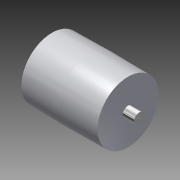
# Autodesk Inventor part: Flexiwheel Roller
Saved by Autodesk Inventor 2014 (Build 180170000, 170)
## iProperties
Created: 2014-02-03
Part Number: Flexiwheel Roller
Material: PPS Plastic
Document SubType Name: Modeling
Designer: Spooner
Density: 1.637 g/cm^3
Appearance: Snow
Author: Spooner
Autodesk Inventor part; units mm, degrees
ref_plane "YZ Plane" through (0, 0, 0) normal (1, 0, 0) x (0, 1, 0)
ref_plane "XZ Plane" through (0, 0, 0) normal (0, 1, 0) x (-1, 0, 0)
ref_plane "XY Plane" through (0, 0, 0) normal (0, 0, 1) x (1, 0, 0)
sketch "Sketch1" plane through (0, 0, 0) normal (0, 0, 1) x (1, 0, 0)
  line L0 (-7.366, 0) -> (7.366, 0)
  line L1 (-7.366, 0) -> (-7.366, 0.8128)
  line L2 (-7.366, 0.8128) -> (-5.6642, 0.8128)
  line L3 (-5.6642, 0.8128) -> (-5.6642, 4.5466)
  line L4 (-5.6642, 4.5466) -> (0, 4.6228)
  line L5 (0, 4.6228) -> (5.6642, 4.5466)
  line L6 (5.6642, 4.5466) -> (5.6642, 0.8128)
  line L7 (5.6642, 0.8128) -> (7.366, 0.8128)
  line L8 (7.366, 0.8128) -> (7.366, 0)
  point P0 (0, 0)
  point P1 (0, 0)
  dimension "d0" = 14.732
  dimension "d1" = 0.8128
  dimension "d2" = 4.6228
  dimension "d3" = 4.5466
  dimension "d4" = 11.3284
  dimension "d5" = 1.7018
  dimension "d6" = 1.7018
  constraints: 18 end point, 3 parallel, 2 horizontal alignment, 2 perpendicular, 1 coincident, 1 collinear, 1 horizontal, 1 midpoint, 1 vertical alignment
  measures "d0" distance of L0.start L0.end
  measures "d1" distance between parallel lines of L0 L2
  measures "d2" distance of point (0, 0) L4.end
  measures "d3" distance from line of L0 L3.end
  measures "d4" distance between parallel lines of L6 L3
  measures "d5" distance from line of L1.end L3
  measures "d6" distance from line of L7.end L6
revolve "Revolution1" add sketch "Sketch1" angle 360 about axis through (-7.366, 0, 0) along (1, 0, 0)
equation "\"d5\" = d6"
body "Solid1"
